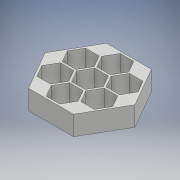
# Autodesk Inventor part: Hexagon pill box
Saved by Autodesk Inventor 2018.2 (Build 222227000, 227)
## iProperties
Created: 2018-03-03
Part Number: Hexagon pill box
Material: Generic
Document SubType Name: Modeling
Designer: Liam McNamee
Density: 1 g/cm^3
Appearance: Default
Author: Liam McNamee
Autodesk Inventor part; units mm, degrees
ref_plane "YZ Plane" through (0, 0, 0) normal (1, 0, 0) x (0, 1, 0)
ref_plane "XZ Plane" through (0, 0, 0) normal (0, 1, 0) x (-1, 0, 0)
ref_plane "XY Plane" through (0, 0, 0) normal (0, 0, 1) x (1, 0, 0)
sketch "Sketch3" plane through (0, 0, 0) normal (0, 0, 1) x (1, 0, 0)
  line L0 (69.282, 0) -> (34.641, -60)
  line L1 (34.641, -60) -> (-34.641, -60)
  line L2 (-34.641, -60) -> (-69.282, 0)
  line L3 (-69.282, 0) -> (-34.641, 60)
  line L4 (-34.641, 60) -> (34.641, 60)
  line L5 (34.641, 60) -> (69.282, 0)
  line L6 (0, 39) -> (33.775, 19.5) construction
  line L7 (33.775, 19.5) -> (33.775, -19.5) construction
  line L8 (33.775, -19.5) -> (0, -39) construction
  line L9 (0, -39) -> (-33.775, -19.5) construction
  line L10 (-33.775, -19.5) -> (-33.775, 19.5) construction
  line L11 (-33.775, 19.5) -> (0, 39) construction
  line L12 (-184.4044, 0) -> (172.1196, 0) construction
  line L13 (0, 140.5486) -> (0, -103.923) construction
  line L14 (20.7846, 39) -> (10.3923, 21)
  line L15 (10.3923, 21) -> (-10.3923, 21)
  line L16 (-10.3923, 21) -> (-20.7846, 39)
  line L17 (-20.7846, 39) -> (-10.3923, 57)
  line L18 (-10.3923, 57) -> (10.3923, 57)
  line L19 (10.3923, 57) -> (20.7846, 39)
  line L20 (-12.9904, 19.5) -> (-23.3827, 1.5)
  line L21 (-23.3827, 37.5) -> (-12.9904, 19.5)
  line L22 (-44.1673, 1.5) -> (-54.5596, 19.5)
  line L23 (-44.1673, 37.5) -> (-23.3827, 37.5)
  line L24 (-54.5596, 19.5) -> (-44.1673, 37.5)
  line L25 (-23.3827, 1.5) -> (-44.1673, 1.5)
  line L26 (-23.3827, -1.5) -> (-12.9904, -19.5)
  line L27 (-44.1673, -1.5) -> (-23.3827, -1.5)
  line L28 (-23.3827, -37.5) -> (-44.1673, -37.5)
  line L29 (-54.5596, -19.5) -> (-44.1673, -1.5)
  line L30 (-44.1673, -37.5) -> (-54.5596, -19.5)
  line L31 (-12.9904, -19.5) -> (-23.3827, -37.5)
  line L32 (-10.3923, -21) -> (10.3923, -21)
  line L33 (-20.7846, -39) -> (-10.3923, -21)
  line L34 (20.7846, -39) -> (10.3923, -57)
  line L35 (-10.3923, -57) -> (-20.7846, -39)
  line L36 (10.3923, -57) -> (-10.3923, -57)
  line L37 (10.3923, -21) -> (20.7846, -39)
  line L38 (12.9904, -19.5) -> (23.3827, -1.5)
  line L39 (23.3827, -37.5) -> (12.9904, -19.5)
  line L40 (44.1673, -1.5) -> (54.5596, -19.5)
  line L41 (44.1673, -37.5) -> (23.3827, -37.5)
  line L42 (54.5596, -19.5) -> (44.1673, -37.5)
  line L43 (23.3827, -1.5) -> (44.1673, -1.5)
  line L44 (23.3827, 1.5) -> (12.9904, 19.5)
  line L45 (44.1673, 1.5) -> (23.3827, 1.5)
  line L46 (23.3827, 37.5) -> (44.1673, 37.5)
  line L47 (54.5596, 19.5) -> (44.1673, 1.5)
  line L48 (44.1673, 37.5) -> (54.5596, 19.5)
  line L49 (12.9904, 19.5) -> (23.3827, 37.5)
  line L50 (-10.3923, 18) -> (10.3923, 18)
  line L51 (10.3923, 18) -> (20.7846, 0)
  line L52 (20.7846, 0) -> (10.3923, -18)
  line L53 (10.3923, -18) -> (-10.3923, -18)
  line L54 (-10.3923, -18) -> (-20.7846, 0)
  line L55 (-20.7846, 0) -> (-10.3923, 18)
  point P0 (0, 0)
  point P1 (0, 0)
  point P2 (0, 0)
  point P3 (-33.775, 19.5)
  point P4 (-33.775, 19.5)
  point P5 (-33.775, -19.5)
  point P6 (-33.775, -19.5)
  point P7 (0, -39)
  point P8 (0, -39)
  point P9 (33.775, -19.5)
  point P10 (33.775, -19.5)
  point P11 (33.775, 19.5)
  point P12 (33.775, 19.5)
  dimension "d58" = 60
  dimension "d59" = 90
  dimension "hex_construct" = 39
  dimension "mini_hex" = 18
  dimension "d65" = 360
  dimension "d69" = 39
  dimension "d74" = 60
  dimension "d75" = 60
  constraints: 112 end point, 8 coincident, 1 horizontal, 1 parallel, 1 vertical, 136 other
  measures "d58" angle of L3 L12
  measures "d59" angle of L10 L12
  measures "hex_construct" distance of L6.end L7.end
  measures "mini_hex" distance from line of L18 L6.start
  measures "d69" distance of L17.end L50.start
  measures "d74" distance from line of L5 point (0, 0)
  measures "d75" angle of L55 L12
sketch "Sketch4" plane through (0, 0, 0) normal (0, 0, 1) x (1, 0, 0)
  line L0 (-34.641, 60) -> (34.641, 60) projected
  line L1 (34.641, 60) -> (69.282, 0) projected
  line L2 (69.282, 0) -> (34.641, -60) projected
  line L3 (34.641, -60) -> (-34.641, -60) projected
  line L4 (-34.641, -60) -> (-69.282, 0) projected
  line L5 (-69.282, 0) -> (-34.641, 60) projected
  line L6 (34.641, 60) -> (69.282, 0)
  line L7 (69.282, 0) -> (34.641, -60)
  line L8 (34.641, -60) -> (-34.641, -60)
  line L9 (-34.641, -60) -> (-69.282, 0)
  line L10 (-69.282, 0) -> (-34.641, 60)
  line L11 (-34.641, 60) -> (34.641, 60)
  point P0 (0, 0)
  point P1 (0, 0)
  constraints: 12 end point, 1 coincident, 13 other
extrude "Extrusion6" add sketch "Sketch4" against normal blind 30
extrude "Extrusion7" cut sketch "Sketch3" against normal blind 27 contours L14 L15 L16 L17 L18 L19 | L20 L25 L22 L24 L23 L21 | L26 L31 L28 L30 L29 L27 | L32 L37 L34 L36 L35 L33 | L38 L43 L40 L42 L41 L39 | L44 L49 L46 L48 L47 L45 | L50 L51 L52 L53 L54 L55
sketch "Sketch5" plane through (0, 0, -30) normal (0, 0, -1) x (-1, 0, 0)
  point P0 (0, 0)
equation "\"wall_thickness\" = 3"
body "Solid2"
